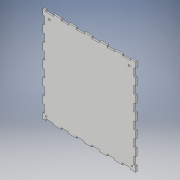
# Autodesk Inventor part: 7 achter plaat
Saved by Autodesk Inventor 2019 (Build 230136000, 136)
## iProperties
Created: 2021-01-22
Part Number: 7 achter plaat
Material: Generic
Document SubType Name: Sheet Metal
Designer: Stefan
Density: 1 g/cm^3
Sheet Metal Rule: Default_mm
Appearance: Default
Author: Stefan
Autodesk Inventor part; units mm, degrees
ref_plane "YZ Plane" through (0, 0, 0) normal (1, 0, 0) x (0, 1, 0)
ref_plane "XZ Plane" through (0, 0, 0) normal (0, 1, 0) x (-1, 0, 0)
ref_plane "XY Plane" through (0, 0, 0) normal (0, 0, 1) x (1, 0, 0)
sketch "Sketch1" plane through (0, 0, 0) normal (0, 0, 1) x (1, 0, 0)
  line L0 (-90.5, -90.5) -> (90.5, -90.5)
  line L1 (90.5, -90.5) -> (90.5, 90.5)
  line L2 (90.5, 90.5) -> (-90.5, 90.5)
  line L3 (-90.5, 90.5) -> (-90.5, -90.5)
  line L4 (-90.5, -90.5) -> (90.5, 90.5) construction
  line L5 (90.5, -90.5) -> (-90.5, 90.5) construction
  point P0 (0, 0)
  dimension "d0" = 181
  dimension "d1" = 181
  constraints: 12 end point, 2 midpoint, 2 parallel, 1 horizontal, 1 perpendicular
  measures "d0" distance of L2.end L1.end
  measures "d1" distance of L1.end L0.end
extrude "Extrusion1" add sketch "Sketch1" along normal blind 3
sketch "Sketch2" plane through (0, 0, 3) normal (0, 0, 1) x (1, 0, 0)
  line L0 (90.5, 90.5) -> (-90.5, 90.5) projected
  line L1 (-90.5, 90.5) -> (-85, 90.5)
  line L2 (-85, 90.5) -> (-85, 93.5)
  line L3 (-85, 93.5) -> (-90.5, 93.5)
  line L4 (-90.5, 93.5) -> (-90.5, 90.5)
  line L5 (80, 90.5) -> (85.5, 90.5)
  line L6 (85.5, 90.5) -> (85.5, 93.5)
  line L7 (85.5, 93.5) -> (80, 93.5)
  line L8 (80, 93.5) -> (80, 90.5)
  line L9 (-90.5, -93.5) -> (-85, -93.5)
  line L10 (-85, -93.5) -> (-85, -90.5)
  line L11 (-85, -90.5) -> (-90.5, -90.5)
  line L12 (-90.5, -90.5) -> (-90.5, -93.5)
  line L13 (80, -93.5) -> (85.5, -93.5)
  line L14 (85.5, -93.5) -> (85.5, -90.5)
  line L15 (85.5, -90.5) -> (80, -90.5)
  line L16 (80, -90.5) -> (80, -93.5)
  line L17 (-70, 90.5) -> (-55, 90.5)
  line L18 (-55, 90.5) -> (-55, 93.5)
  line L19 (-55, 93.5) -> (-70, 93.5)
  line L20 (-70, 93.5) -> (-70, 90.5)
  line L21 (-25, 90.5) -> (-25, 93.5)
  line L22 (-40, 90.5) -> (-25, 90.5)
  line L23 (-25, 93.5) -> (-40, 93.5)
  line L24 (-40, 93.5) -> (-40, 90.5)
  line L25 (5, 90.5) -> (5, 93.5)
  line L26 (-10, 90.5) -> (5, 90.5)
  line L27 (5, 93.5) -> (-10, 93.5)
  line L28 (-10, 93.5) -> (-10, 90.5)
  line L29 (35, 90.5) -> (35, 93.5)
  line L30 (20, 90.5) -> (35, 90.5)
  line L31 (35, 93.5) -> (20, 93.5)
  line L32 (20, 93.5) -> (20, 90.5)
  line L33 (65, 90.5) -> (65, 93.5)
  line L34 (50, 90.5) -> (65, 90.5)
  line L35 (65, 93.5) -> (50, 93.5)
  line L36 (50, 93.5) -> (50, 90.5)
  line L37 (-55, -93.5) -> (-55, -90.5)
  line L38 (-70, -93.5) -> (-55, -93.5)
  line L39 (-55, -90.5) -> (-70, -90.5)
  line L40 (-70, -90.5) -> (-70, -93.5)
  line L41 (-25, -93.5) -> (-25, -90.5)
  line L42 (-40, -93.5) -> (-25, -93.5)
  line L43 (-25, -90.5) -> (-40, -90.5)
  line L44 (-40, -90.5) -> (-40, -93.5)
  line L45 (5, -93.5) -> (5, -90.5)
  line L46 (-10, -93.5) -> (5, -93.5)
  line L47 (5, -90.5) -> (-10, -90.5)
  line L48 (-10, -90.5) -> (-10, -93.5)
  line L49 (35, -93.5) -> (35, -90.5)
  line L50 (20, -93.5) -> (35, -93.5)
  line L51 (35, -90.5) -> (20, -90.5)
  line L52 (20, -90.5) -> (20, -93.5)
  line L53 (65, -93.5) -> (65, -90.5)
  line L54 (50, -93.5) -> (65, -93.5)
  line L55 (65, -90.5) -> (50, -90.5)
  line L56 (50, -90.5) -> (50, -93.5)
  point P0 (0, 0)
  dimension "d4" = 5.5
  dimension "d5" = 3
  dimension "d8" = 170.5
  dimension "d11" = 184
  dimension "d14" = 15
  dimension "d15" = 3
  dimension "d16" = 15
  dimension "d19" = 30
  dimension "d22" = 184
  constraints: 112 end point, 4 horizontal, 4 parallel, 3 collinear, 2 perpendicular, 2 vertical, 1 point on line, 93 other
  measures "d4" distance of L3.end L2.end
  measures "d5" distance of L2.end L1.end
  measures "d8" distance of L2.end L6.end
  measures "d11" distance of L2.end L10.end
  measures "d14" distance of L19.end L18.end
  measures "d15" distance of L18.end L17.end
  measures "d16" distance between parallel lines of L20 L2
  measures "d19" distance of L17.end L21.start
  measures "d22" distance of L17.end L37.start
extrude "Extrusion2" add sketch "Sketch2" against normal blind 3
sketch "Sketch3" plane through (0, 0, 3) normal (0, 0, 1) x (1, 0, 0)
  line L0 (-90.5, 93.5) -> (-90.5, -93.5) projected
  line L1 (-90.5, 82.5) -> (-87.5, 82.5)
  line L2 (-87.5, 82.5) -> (-87.5, 67.5)
  line L3 (-87.5, 67.5) -> (-90.5, 67.5)
  line L4 (-90.5, 67.5) -> (-90.5, 82.5)
  line L5 (-85, 93.5) -> (-90.5, 93.5) projected
  line L6 (-90.5, 52.5) -> (-87.5, 52.5)
  line L7 (-87.5, 52.5) -> (-87.5, 37.5)
  line L8 (-87.5, 37.5) -> (-90.5, 37.5)
  line L9 (-90.5, 37.5) -> (-90.5, 52.5)
  line L10 (-90.5, 22.5) -> (-87.5, 22.5)
  line L11 (-87.5, 22.5) -> (-87.5, 7.5)
  line L12 (-87.5, 7.5) -> (-90.5, 7.5)
  line L13 (-90.5, 7.5) -> (-90.5, 22.5)
  line L14 (-90.5, -7.5) -> (-87.5, -7.5)
  line L15 (-87.5, -7.5) -> (-87.5, -22.5)
  line L16 (-87.5, -22.5) -> (-90.5, -22.5)
  line L17 (-90.5, -22.5) -> (-90.5, -7.5)
  line L18 (-90.5, -37.5) -> (-87.5, -37.5)
  line L19 (-87.5, -37.5) -> (-87.5, -52.5)
  line L20 (-87.5, -52.5) -> (-90.5, -52.5)
  line L21 (-90.5, -52.5) -> (-90.5, -37.5)
  line L22 (-90.5, -67.5) -> (-87.5, -67.5)
  line L23 (-87.5, -67.5) -> (-87.5, -82.5)
  line L24 (-87.5, -82.5) -> (-90.5, -82.5)
  line L25 (-90.5, -82.5) -> (-90.5, -67.5)
  line L26 (87.5, 82.5) -> (90.5, 82.5)
  line L27 (90.5, 82.5) -> (90.5, 67.5)
  line L28 (90.5, 67.5) -> (87.5, 67.5)
  line L29 (87.5, 67.5) -> (87.5, 82.5)
  line L30 (87.5, 52.5) -> (90.5, 52.5)
  line L31 (90.5, 52.5) -> (90.5, 37.5)
  line L32 (90.5, 37.5) -> (87.5, 37.5)
  line L33 (87.5, 37.5) -> (87.5, 52.5)
  line L34 (87.5, 22.5) -> (90.5, 22.5)
  line L35 (90.5, 22.5) -> (90.5, 7.5)
  line L36 (90.5, 7.5) -> (87.5, 7.5)
  line L37 (87.5, 7.5) -> (87.5, 22.5)
  line L38 (87.5, -7.5) -> (90.5, -7.5)
  line L39 (90.5, -7.5) -> (90.5, -22.5)
  line L40 (90.5, -22.5) -> (87.5, -22.5)
  line L41 (87.5, -22.5) -> (87.5, -7.5)
  line L42 (87.5, -37.5) -> (90.5, -37.5)
  line L43 (90.5, -37.5) -> (90.5, -52.5)
  line L44 (90.5, -52.5) -> (87.5, -52.5)
  line L45 (87.5, -52.5) -> (87.5, -37.5)
  line L46 (87.5, -67.5) -> (90.5, -67.5)
  line L47 (90.5, -67.5) -> (90.5, -82.5)
  line L48 (90.5, -82.5) -> (87.5, -82.5)
  line L49 (87.5, -82.5) -> (87.5, -67.5)
  point P0 (0, 0)
  dimension "d27" = 3
  dimension "d28" = 15
  dimension "d29" = 11
  dimension "d32" = 30
  dimension "d35" = 178
  constraints: 96 end point, 2 horizontal, 2 parallel, 1 perpendicular, 1 point on line, 1 vertical, 88 other
  measures "d27" distance of L2.end L3.end
  measures "d28" distance of L1.end L2.end
  measures "d29" distance between parallel lines of L5 L1
  measures "d32" distance of L1.start L6.start
  measures "d35" distance of L1.start L26.start
extrude "Extrusion3" cut sketch "Sketch3" against normal blind 3
sketch "Sketch4" plane through (0, 0, 3) normal (0, 0, 1) x (1, 0, 0)
  line L0 (80, 93.5) -> (85.5, 93.5) projected
  line L1 (90.5, 90.5) -> (85.5, 90.5) projected
  line L2 (85.5, 93.5) -> (90.5, 93.5)
  line L3 (90.5, 93.5) -> (90.5, 90.5)
  line L4 (90.5, 90.5) -> (85.5, 90.5)
  line L5 (85.5, 90.5) -> (85.5, 93.5)
  line L6 (85.5, -90.5) -> (90.5, -90.5) projected
  line L7 (85.5, -90.5) -> (90.5, -90.5)
  line L8 (90.5, -90.5) -> (90.5, -93.5)
  line L9 (90.5, -93.5) -> (85.5, -93.5)
  line L10 (85.5, -93.5) -> (85.5, -90.5)
  point P0 (0, 0)
  dimension "d40" = 184
  constraints: 16 end point, 4 parallel, 2 horizontal, 2 perpendicular, 1 point on line
  measures "d40" distance between parallel lines of L1 L9
extrude "Extrusion4" add sketch "Sketch4" against normal blind 3
sketch "Sketch5" plane through (0, 0, 3) normal (0, 0, 1) x (1, 0, 0)
  circle A0 centre (-84, -86) radius 1.5
  circle A1 centre (84, -86) radius 1.5
  line L0 (90.5, -82.5) -> (90.5, -93.5) projected
  line L1 (90.5, -93.5) -> (80, -93.5) projected
  line L2 (-85, -93.5) -> (-90.5, -93.5) projected
  line L3 (-90.5, -82.5) -> (-90.5, -93.5) projected
  point P0 (0, 0)
  dimension "d43" = 3
  dimension "d44" = 3
  dimension "d45" = 6.5
  dimension "d46" = 7.5
  dimension "d47" = 7.5
  dimension "d48" = 6.5
  constraints: 2 centre point
  measures "d43" diameter of A0
  measures "d44" diameter of A1
  measures "d45" distance from line of L0 A1.centre
  measures "d46" distance from line of L1 A1.centre
  measures "d47" distance from line of L2 A0.centre
  measures "d48" distance from line of A0.centre L3
extrude "Extrusion5" cut sketch "Sketch5" against normal blind 10
sketch "Sketch6" plane through (0, 0, 3) normal (0, 0, 1) x (1, 0, 0)
  circle A0 centre (-78, 81) radius 2
  circle A1 centre (78, 81) radius 2
  line L0 (-87.5, 82.5) -> (-87.5, 67.5) projected
  line L1 (-70, 90.5) -> (-85, 90.5) projected
  line L2 (80, 90.5) -> (65, 90.5) projected
  line L3 (87.5, 67.5) -> (87.5, 82.5) projected
  point P0 (0, 0)
  dimension "d51" = 4
  dimension "d52" = 4
  dimension "d53" = 9.5
  dimension "d54" = 9.5
  dimension "d55" = 9.5
  dimension "d56" = 9.5
  constraints: 2 centre point
  measures "d51" diameter of A0
  measures "d52" diameter of A1
  measures "d53" distance from line of L0 A0.centre
  measures "d54" distance from line of L1 A0.centre
  measures "d55" distance from line of L2 A1.centre
  measures "d56" distance from line of L3 A1.centre
extrude "Extrusion6" cut sketch "Sketch6" against normal blind 10
equation "\"d47\" = d46"
equation "\"d48\" = d45"
equation "\"BendRadius\" = Thickness"
equation "\"BendReliefWidth\" = Thickness"
equation "\"BendReliefDepth\" = 0.5 * Thickness"
equation "\"CornerReliefSize\" = 4 * Thickness"
equation "\"MinimumRemnant\" = 2 * Thickness"
equation "\"TransitionRadius\" = BendRadius"
equation "\"JacobiRadiusSize\" = BendRadius"
equation "\"GapSize\" = Thickness"
equation "\"Thickness\" = 0.5"
body "Solid1"
